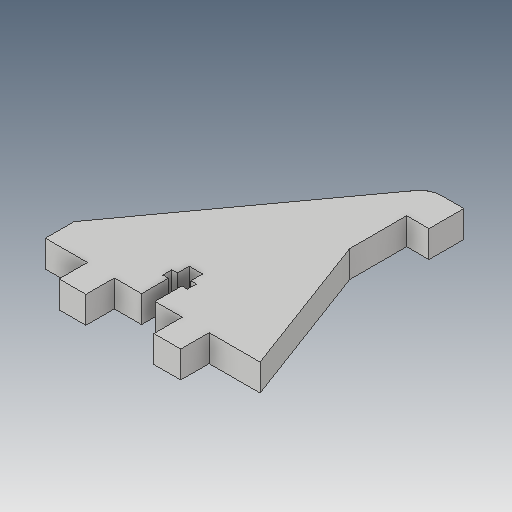
# Autodesk Inventor part: Z Motor Mount Brace
Saved by Autodesk Inventor 2017 (Build 210142000, 142)
## iProperties
Created: 2016-07-25
Part Number: Z Motor Mount Brace
Material: Generic
Document SubType Name: Modeling
Designer: User
Density: 1 g/cm^3
Appearance: Default
Mass: 8.3381 g
Surface Area: 41.5941 cm^2
Volume: 8.3381 cm^3
Author: User
Autodesk Inventor part; units mm, degrees
ref_plane "YZ Plane" through (0, 0, 0) normal (1, 0, 0) x (0, 1, 0)
ref_plane "XZ Plane" through (0, 0, 0) normal (0, 1, 0) x (-1, 0, 0)
ref_plane "XY Plane" through (0, 0, 0) normal (0, 0, 1) x (1, 0, 0)
sketch "Sketch1" plane through (0, 0, 0) normal (0, 1, 0) x (-1, 0, 0)
  line L0 (180.5524, 781.9255) -> (180.551, 788.2755)
  line L1 (180.551, 788.2755) -> (174.551, 788.2742)
  line L2 (174.551, 788.2742) -> (174.5524, 781.9242)
  line L3 (174.5524, 781.9242) -> (168.4524, 781.9229)
  line L4 (168.4524, 781.9229) -> (168.4537, 775.9228)
  line L5 (168.4537, 775.9228) -> (169.7037, 775.9231)
  line L6 (169.7037, 775.9231) -> (169.7042, 773.9231)
  line L7 (169.7042, 773.9231) -> (168.4542, 773.9229)
  line L8 (168.4542, 773.9229) -> (168.4547, 771.2728)
  line L9 (168.4547, 771.2728) -> (165.4547, 771.2722)
  line L10 (165.4547, 771.2722) -> (165.4541, 773.9222)
  line L11 (165.4541, 773.9222) -> (164.2041, 773.9219)
  line L12 (164.2041, 773.9219) -> (164.2037, 775.9219)
  line L13 (164.2037, 775.9219) -> (165.4537, 775.9222)
  line L14 (165.4537, 775.9222) -> (165.4524, 781.9222)
  line L15 (165.4524, 781.9222) -> (159.3524, 781.9209)
  line L16 (159.3524, 781.9209) -> (159.351, 788.2709)
  line L17 (159.351, 788.2709) -> (153.351, 788.2696)
  line L18 (153.351, 788.2696) -> (153.3524, 781.9196)
  line L19 (153.3524, 781.9196) -> (141.9524, 781.9171)
  line L20 (141.9524, 781.9171) -> (153.9094, 749.9197)
  line L21 (153.9094, 749.9197) -> (153.9122, 737.1696)
  line L22 (153.9122, 737.1696) -> (148.9122, 737.1685)
  line L23 (148.9122, 737.1685) -> (148.9139, 729.3686)
  line L24 (148.9139, 729.3686) -> (153.9139, 729.3697)
  line L25 (153.9139, 729.3697) -> (154.0889, 729.3947)
  line L26 (154.0889, 729.3947) -> (155.1888, 729.545)
  line L27 (155.1888, 729.545) -> (156.4138, 730.0452)
  line L28 (156.4138, 730.0452) -> (157.4386, 730.8204)
  line L29 (157.4386, 730.8204) -> (158.2386, 731.8705)
  line L30 (158.2386, 731.8705) -> (189.9642, 775.495)
  line L31 (189.9642, 775.495) -> (189.9628, 781.9276)
  line L32 (189.9628, 781.9276) -> (180.5524, 781.9255)
  point P0 (0, 0)
  constraints: 66 end point, 10 parallel, 7 perpendicular
extrude "Extrusion1" add sketch "Sketch1" along normal blind 6
body "Solid1"
